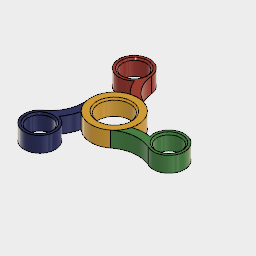
fusion (Autodesk Fusion 360 design; units mm, degrees)
Autodesk Fusion 360 part; units mm, degrees
sketch "Sketch3" plane through (0, 0, 0) normal (0, 0, 1) x (1, 0, 0)
  circle A0 centre (0, 0) radius 15
  circle A1 centre (35, 0) radius 10
  arc A2 (30.9044, -9.1228) -> (9.2793, -11.7854) centre (22.2903, -28.3102) ccw
  circle A3 centre (0, 0) radius 10
  line L0 (1.75, 0) -> (22.5, 0) construction
  circle A4 centre (35, 0) radius 7.5
  arc A5 (25.3315, -2.5534) -> (14.5741, -3.549) centre (22.2903, -28.3102) ccw
  arc A6 (-10.4544, 23.2144) -> (-4.2136, 14.396) centre (13.3722, 33.4591) ccw
  arc A7 (-7.5516, 31.3254) -> (5.5668, 13.9288) centre (13.3722, 33.4591) ccw
  circle A8 centre (-17.5, 30.3109) radius 10
  circle A9 centre (-17.5, 30.3109) radius 7.5
  arc A10 (-14.8771, -20.661) -> (-10.3605, -10.8471) centre (-35.6626, -5.1489) ccw
  arc A11 (-23.3528, -22.2026) -> (-14.8461, -2.1434) centre (-35.6626, -5.1489) ccw
  circle A12 centre (-17.5, -30.3109) radius 10
  circle A13 centre (-17.5, -30.3109) radius 7.5
  dimension "d22" = 30
  dimension "d25" = 20
  dimension "d34" = 20
  dimension "d36" = 15
  dimension "d40" = 360
  dimension "d49" = 35
  measures "d22" diameter of A0
  measures "d25" diameter of A1
  measures "d34" diameter of A3
  measures "d36" diameter of A4
  measures "d49" distance of A0.centre A1.centre
extrude "Extrude5" add sketch "Sketch3" along normal blind 10 contours A0 makes body 1
extrude "Extrude6" add sketch "Sketch3" along normal blind 10 separate body contours A0 A6 A7 A8 | A0 A1 A2 A5 | A8 | A1 | A0 A10 A11 A12 | A12 makes body 2 at (25.1251, -1.5768, 3.3333) makes body 3 at (-23.68, 22.4491, 6.6667) makes body 4 at (-24.132, -22.8265, 6.6667)
chamfer "Chamfer1" distance 1 angle 45 4 edges at (28.0075, 2.7121, 10) (-9.3233, 3.6162, 10) (-24.4925, 33.023, 10) (-24.4925, -27.5988, 10) on bodies 1 2 3 4
